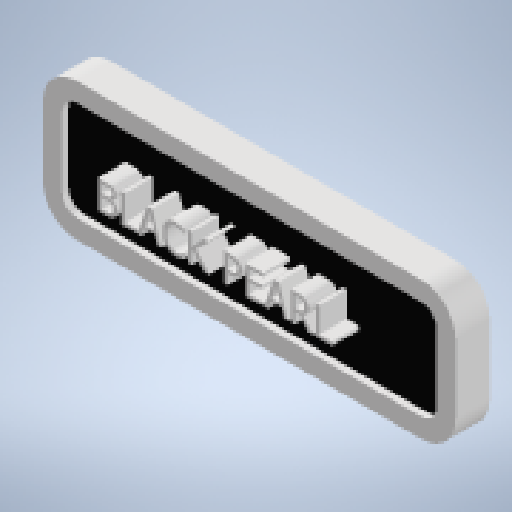
# Autodesk Inventor part: name of ship
Saved by Autodesk Inventor 2024.1 (Build 281209000, 209)
## iProperties
Created: 2023-10-19
Part Number: name of ship
Material: Generic
Document SubType Name: Modeling
Designer: Manaswi
Density: 1 g/cm^3
Appearance: Default
Author: Manaswi
Autodesk Inventor part; units mm, degrees
ref_plane "YZ Plane" through (0, 0, 0) normal (1, 0, 0) x (0, 1, 0)
ref_plane "XZ Plane" through (0, 0, 0) normal (0, 1, 0) x (-1, 0, 0)
ref_plane "XY Plane" through (0, 0, 0) normal (0, 0, 1) x (1, 0, 0)
sketch "Sketch1" plane through (0, 0, 0) normal (0, 0, 1) x (1, 0, 0)
  line L0 (0, 0) -> (6000, 0)
  line L1 (6000, 0) -> (6000, 2000)
  line L2 (6000, 2000) -> (0, 2000)
  line L3 (0, 2000) -> (0, 0)
  dimension "d0" = 2000
  dimension "d1" = 6000
  constraints: 8 end point, 3 perpendicular, 1 horizontal
  measures "d0" distance of L0.start L2.end
  measures "d1" distance of L2.end L1.end
extrude "Extrusion1" add sketch "Sketch1" along normal blind 500
fillet "Fillet1" radius 500 4 edges at (6000, 2000, 250) (6000, 0, 250) (0, 2000, 250) (0, 0, 250)
sketch "Sketch2" plane through (0, 0, 500) normal (0, 0, 1) x (1, 0, 0)
  arc A0 (0, 500) -> (500, 0) centre (500, 500) ccw projected
  line L0 (500, 0) -> (5500, 0) projected
  arc A1 (5500, 0) -> (6000, 500) centre (5500, 500) ccw projected
  line L1 (6000, 500) -> (6000, 1500) projected
  arc A2 (6000, 1500) -> (5500, 2000) centre (5500, 1500) ccw projected
  line L2 (5500, 2000) -> (500, 2000) projected
  arc A3 (500, 2000) -> (0, 1500) centre (500, 1500) ccw projected
  line L3 (0, 1500) -> (0, 500) projected
  line L4 (500, 1720.5162) -> (5500, 1720.5162)
  arc A4 (5720.5162, 1500) -> (5500, 1720.5162) centre (5500, 1500) ccw
  line L5 (5720.5162, 1500) -> (5720.5162, 500)
  arc A5 (5500, 279.4838) -> (5720.5162, 500) centre (5500, 500) ccw
  line L6 (5500, 279.4838) -> (500, 279.4838)
  arc A6 (279.4838, 500) -> (500, 279.4838) centre (500, 500) ccw
  line L7 (279.4838, 500) -> (279.4838, 1500)
  arc A7 (500, 1720.5162) -> (279.4838, 1500) centre (500, 1500) ccw
  point P0 (0, 0)
  constraints: 8 end point, 8 point on circle, 4 centre point, 7 other
extrude "Extrusion2" cut sketch "Sketch2" against normal blind 100 contours L4 A4 L5 A5 L6 A6 L7 A7
sketch "Sketch3" plane through (0, 0, 400) normal (0, 0, 1) x (1, 0, 0)
  line L0 (1060.4383, 1242.6804) -> (4504.2158, 1242.6804) construction
  line L1 (4504.2158, 1242.6804) -> (4504.2158, 811.7024) construction
  line L2 (4504.2158, 811.7024) -> (1060.4383, 811.7024) construction
  line L3 (1060.4383, 811.7024) -> (1060.4383, 1242.6804) construction
  spline S0 degree 2 poles (1384.8522, 946.931) (1384.8522, 915.906) (1361.2462, 868.3567) (1341.6869, 852.8442) knots 0 0 0 1 2 2 2
  spline S1 degree 2 poles (1341.6869, 852.8442) (1318.0809, 834.6339) (1264.4616, 819.1214) (1221.9708, 819.1214) knots 0 0 0 1 2 2 2
  line L4 (1221.9708, 819.1214) -> (1102.5919, 819.1214)
  line L5 (1102.5919, 819.1214) -> (1102.5919, 1235.2614)
  line L6 (1102.5919, 1235.2614) -> (1212.8656, 1235.2614)
  spline S2 degree 2 poles (1212.8656, 1235.2614) (1257.3798, 1235.2614) (1301.894, 1229.5285) (1322.1277, 1218.3999) knots 0 0 0 1 2 2 2
  spline S3 degree 2 poles (1322.1277, 1218.3999) (1344.722, 1206.5969) (1365.2929, 1167.8157) (1365.2929, 1141.5118) knots 0 0 0 1 2 2 2
  spline S4 degree 2 poles (1365.2929, 1141.5118) (1365.2929, 1112.173) (1334.2679, 1065.6354) (1306.9524, 1052.4835) knots 0 0 0 1 2 2 2
  line L7 (1306.9524, 1052.4835) -> (1306.9524, 1050.4601)
  spline S5 degree 2 poles (1306.9524, 1050.4601) (1344.0475, 1040.3433) (1384.8522, 986.7239) (1384.8522, 946.931) knots 0 0 0 1 2 2 2
  spline S6 degree 2 poles (1327.1861, 944.5704) (1327.1861, 968.1764) (1313.697, 998.5269) (1293.4633, 1009.3183) knots 0 0 0 1 2 2 2
  spline S7 degree 2 poles (1293.4633, 1009.3183) (1280.3113, 1016.0628) (1249.2863, 1020.1096) (1220.6219, 1020.1096) knots 0 0 0 1 2 2 2
  line L8 (1220.6219, 1020.1096) -> (1157.8974, 1020.1096)
  line L9 (1157.8974, 1020.1096) -> (1157.8974, 866.3334)
  line L10 (1157.8974, 866.3334) -> (1202.7488, 866.3334)
  spline S8 degree 2 poles (1202.7488, 866.3334) (1239.1695, 866.3334) (1280.9858, 873.0779) (1297.1728, 883.8693) knots 0 0 0 1 2 2 2
  spline S9 degree 2 poles (1297.1728, 883.8693) (1312.6853, 894.9978) (1327.1861, 922.6505) (1327.1861, 944.5704) knots 0 0 0 1 2 2 2
  spline S10 degree 2 poles (1307.6268, 1133.7556) (1307.6268, 1148.5936) (1297.51, 1170.8507) (1286.3815, 1177.2581) knots 0 0 0 1 2 2 2
  spline S11 degree 2 poles (1286.3815, 1177.2581) (1272.8923, 1184.6771) (1240.1811, 1188.0494) (1210.8423, 1188.0494) knots 0 0 0 1 2 2 2
  line L11 (1210.8423, 1188.0494) -> (1157.8974, 1188.0494)
  line L12 (1157.8974, 1188.0494) -> (1157.8974, 1066.3099)
  line L13 (1157.8974, 1066.3099) -> (1220.6219, 1066.3099)
  spline S12 degree 2 poles (1220.6219, 1066.3099) (1246.5885, 1066.3099) (1271.2062, 1071.7055) (1284.3581, 1080.1362) knots 0 0 0 1 2 2 2
  spline S13 degree 2 poles (1284.3581, 1080.1362) (1297.1728, 1088.2297) (1307.6268, 1114.1963) (1307.6268, 1133.7556) knots 0 0 0 1 2 2 2
  line L14 (1680.9388, 819.1214) -> (1439.8204, 819.1214)
  line L15 (1439.8204, 819.1214) -> (1439.8204, 1235.2614)
  line L16 (1439.8204, 1235.2614) -> (1495.1259, 1235.2614)
  line L17 (1495.1259, 1235.2614) -> (1495.1259, 868.3567)
  line L18 (1495.1259, 868.3567) -> (1680.9388, 868.3567)
  line L19 (1680.9388, 868.3567) -> (1680.9388, 819.1214)
  line L20 (1679.5899, 819.1214) -> (1819.877, 1235.2614)
  line L21 (1819.877, 1235.2614) -> (1887.9971, 1235.2614)
  line L22 (1887.9971, 1235.2614) -> (2028.2842, 819.1214)
  line L23 (2028.2842, 819.1214) -> (1969.9436, 819.1214)
  line L24 (1969.9436, 819.1214) -> (1932.1741, 935.4652)
  line L25 (1932.1741, 935.4652) -> (1773.3394, 935.4652)
  line L26 (1773.3394, 935.4652) -> (1735.5698, 819.1214)
  line L27 (1735.5698, 819.1214) -> (1679.5899, 819.1214)
  line L28 (1916.9988, 982.6772) -> (1852.5881, 1178.607)
  line L29 (1852.5881, 1178.607) -> (1788.5147, 982.6772)
  line L30 (1788.5147, 982.6772) -> (1916.9988, 982.6772)
  spline S14 degree 2 poles (2230.2841, 811.7024) (2189.8166, 811.7024) (2121.3592, 839.0179) (2096.4043, 866.3334) knots 0 0 0 1 2 2 2
  spline S15 degree 2 poles (2096.4043, 866.3334) (2071.4494, 893.3117) (2044.1339, 974.2465) (2044.1339, 1026.8541) knots 0 0 0 1 2 2 2
  spline S16 degree 2 poles (2044.1339, 1026.8541) (2044.1339, 1079.1246) (2070.775, 1156.6871) (2096.0671, 1185.3515) knots 0 0 0 1 2 2 2
  spline S17 degree 2 poles (2096.0671, 1185.3515) (2121.022, 1213.3415) (2189.1422, 1242.6804) (2231.2957, 1242.6804) knots 0 0 0 1 2 2 2
  spline S18 degree 2 poles (2231.2957, 1242.6804) (2252.2039, 1242.6804) (2288.9618, 1236.6103) (2304.4743, 1231.8891) knots 0 0 0 1 2 2 2
  spline S19 degree 2 poles (2304.4743, 1231.8891) (2317.9635, 1227.5051) (2345.9534, 1215.0277) (2359.7798, 1207.6086) knots 0 0 0 1 2 2 2
  line L31 (2359.7798, 1207.6086) -> (2359.7798, 1140.8374)
  line L32 (2359.7798, 1140.8374) -> (2355.3958, 1140.8374)
  spline S20 degree 2 poles (2355.3958, 1140.8374) (2347.9768, 1147.5819) (2325.0453, 1166.4667) (2308.5211, 1175.5719) knots 0 0 0 1 2 2 2
  spline S21 degree 2 poles (2308.5211, 1175.5719) (2292.6713, 1184.3399) (2255.239, 1195.4684) (2230.9585, 1195.4684) knots 0 0 0 1 2 2 2
  spline S22 degree 2 poles (2230.9585, 1195.4684) (2204.3175, 1195.4684) (2156.7682, 1173.5485) (2138.8951, 1152.6404) knots 0 0 0 1 2 2 2
  spline S23 degree 2 poles (2138.8951, 1152.6404) (2121.3592, 1131.395) (2101.8, 1066.9843) (2101.8, 1026.8541) knots 0 0 0 1 2 2 2
  spline S24 degree 2 poles (2101.8, 1026.8541) (2101.8, 984.0261) (2122.3709, 922.3133) (2140.244, 901.0679) knots 0 0 0 1 2 2 2
  spline S25 degree 2 poles (2140.244, 901.0679) (2157.7799, 880.497) (2204.6547, 859.5888) (2230.9585, 859.5888) knots 0 0 0 1 2 2 2
  spline S26 degree 2 poles (2230.9585, 859.5888) (2254.9017, 859.5888) (2295.7064, 871.3918) (2311.5561, 880.1597) knots 0 0 0 1 2 2 2
  spline S27 degree 2 poles (2311.5561, 880.1597) (2326.7314, 888.9277) (2349.3257, 907.138) (2355.7331, 913.5454) knots 0 0 0 1 2 2 2
  line L33 (2355.7331, 913.5454) -> (2359.7798, 913.5454)
  line L34 (2359.7798, 913.5454) -> (2359.7798, 847.4486)
  spline S28 degree 2 poles (2359.7798, 847.4486) (2345.9534, 841.0412) (2321.673, 829.2382) (2304.4743, 823.8426) knots 0 0 0 1 2 2 2
  spline S29 degree 2 poles (2304.4743, 823.8426) (2286.264, 817.7725) (2255.239, 811.7024) (2230.2841, 811.7024) knots 0 0 0 1 2 2 2
  line L35 (2714.8814, 819.1214) -> (2643.0518, 819.1214)
  line L36 (2643.0518, 819.1214) -> (2490.9617, 1012.6905)
  line L37 (2490.9617, 1012.6905) -> (2466.6812, 985.375)
  line L38 (2466.6812, 985.375) -> (2466.6812, 819.1214)
  line L39 (2466.6812, 819.1214) -> (2411.3758, 819.1214)
  line L40 (2411.3758, 819.1214) -> (2411.3758, 1235.2614)
  line L41 (2411.3758, 1235.2614) -> (2466.6812, 1235.2614)
  line L42 (2466.6812, 1235.2614) -> (2466.6812, 1044.0528)
  line L43 (2466.6812, 1044.0528) -> (2637.3189, 1235.2614)
  line L44 (2637.3189, 1235.2614) -> (2704.7646, 1235.2614)
  line L45 (2704.7646, 1235.2614) -> (2532.4408, 1049.4485)
  line L46 (2532.4408, 1049.4485) -> (2714.8814, 819.1214)
  spline S30 degree 2 poles (3189.6992, 1109.8124) (3189.6992, 1082.8341) (3170.4771, 1034.2732) (3153.2785, 1017.4117) knots 0 0 0 1 2 2 2
  spline S31 degree 2 poles (3153.2785, 1017.4117) (3131.6959, 996.1663) (3073.3553, 974.2465) (3028.8412, 974.2465) knots 0 0 0 1 2 2 2
  line L47 (3028.8412, 974.2465) -> (2981.9664, 974.2465)
  line L48 (2981.9664, 974.2465) -> (2981.9664, 819.1214)
  line L49 (2981.9664, 819.1214) -> (2926.6609, 819.1214)
  line L50 (2926.6609, 819.1214) -> (2926.6609, 1235.2614)
  line L51 (2926.6609, 1235.2614) -> (3031.2018, 1235.2614)
  spline S32 degree 2 poles (3031.2018, 1235.2614) (3068.2969, 1235.2614) (3120.2301, 1223.1211) (3140.1266, 1209.2948) knots 0 0 0 1 2 2 2
  spline S33 degree 2 poles (3140.1266, 1209.2948) (3163.3954, 1193.445) (3189.6992, 1144.5469) (3189.6992, 1109.8124) knots 0 0 0 1 2 2 2
  spline S34 degree 2 poles (3132.0331, 1108.1262) (3132.0331, 1129.7088) (3117.195, 1161.4083) (3102.0198, 1171.5252) knots 0 0 0 1 2 2 2
  spline S35 degree 2 poles (3102.0198, 1171.5252) (3088.8678, 1180.2931) (3053.7961, 1187.3749) (3027.8295, 1187.3749) knots 0 0 0 1 2 2 2
  line L52 (3027.8295, 1187.3749) -> (2981.9664, 1187.3749)
  line L53 (2981.9664, 1187.3749) -> (2981.9664, 1021.4585)
  line L54 (2981.9664, 1021.4585) -> (3019.736, 1021.4585)
  spline S36 degree 2 poles (3019.736, 1021.4585) (3053.4589, 1021.4585) (3094.938, 1032.2498) (3108.4271, 1046.4134) knots 0 0 0 1 2 2 2
  spline S37 degree 2 poles (3108.4271, 1046.4134) (3120.9046, 1058.8909) (3132.0331, 1088.2297) (3132.0331, 1108.1262) knots 0 0 0 1 2 2 2
  line L55 (3242.3068, 819.1214) -> (3242.3068, 1235.2614)
  line L56 (3242.3068, 1235.2614) -> (3502.6472, 1235.2614)
  line L57 (3502.6472, 1235.2614) -> (3502.6472, 1186.026)
  line L58 (3502.6472, 1186.026) -> (3297.6123, 1186.026)
  line L59 (3297.6123, 1186.026) -> (3297.6123, 1072.0428)
  line L60 (3297.6123, 1072.0428) -> (3488.8209, 1072.0428)
  line L61 (3488.8209, 1072.0428) -> (3488.8209, 1022.8074)
  line L62 (3488.8209, 1022.8074) -> (3297.6123, 1022.8074)
  line L63 (3297.6123, 1022.8074) -> (3297.6123, 868.3567)
  line L64 (3297.6123, 868.3567) -> (3502.6472, 868.3567)
  line L65 (3502.6472, 868.3567) -> (3502.6472, 819.1214)
  line L66 (3502.6472, 819.1214) -> (3242.3068, 819.1214)
  line L67 (3518.497, 819.1214) -> (3658.784, 1235.2614)
  line L68 (3658.784, 1235.2614) -> (3726.9042, 1235.2614)
  line L69 (3726.9042, 1235.2614) -> (3867.1913, 819.1214)
  line L70 (3867.1913, 819.1214) -> (3808.8507, 819.1214)
  line L71 (3808.8507, 819.1214) -> (3771.0811, 935.4652)
  line L72 (3771.0811, 935.4652) -> (3612.2465, 935.4652)
  line L73 (3612.2465, 935.4652) -> (3574.4769, 819.1214)
  line L74 (3574.4769, 819.1214) -> (3518.497, 819.1214)
  line L75 (3755.9058, 982.6772) -> (3691.4952, 1178.607)
  line L76 (3691.4952, 1178.607) -> (3627.4218, 982.6772)
  line L77 (3627.4218, 982.6772) -> (3755.9058, 982.6772)
  line L78 (4228.7002, 819.1214) -> (4156.8705, 819.1214)
  line L79 (4156.8705, 819.1214) -> (4025.3514, 984.7006)
  line L80 (4025.3514, 984.7006) -> (3961.9525, 984.7006)
  line L81 (3961.9525, 984.7006) -> (3961.9525, 819.1214)
  line L82 (3961.9525, 819.1214) -> (3906.647, 819.1214)
  line L83 (3906.647, 819.1214) -> (3906.647, 1235.2614)
  line L84 (3906.647, 1235.2614) -> (4013.8857, 1235.2614)
  spline S38 degree 2 poles (4013.8857, 1235.2614) (4049.6319, 1235.2614) (4097.8556, 1227.5051) (4119.7754, 1213.3415) knots 0 0 0 1 2 2 2
  spline S39 degree 2 poles (4119.7754, 1213.3415) (4141.6953, 1199.1779) (4166.9874, 1155.001) (4166.9874, 1122.2898) knots 0 0 0 1 2 2 2
  spline S40 degree 2 poles (4166.9874, 1122.2898) (4166.9874, 1076.764) (4120.4499, 1015.0511) (4080.6569, 1000.2131) knots 0 0 0 1 2 2 2
  line L85 (4080.6569, 1000.2131) -> (4228.7002, 819.1214)
  spline S41 degree 2 poles (4109.3213, 1117.9058) (4109.3213, 1136.1162) (4096.5066, 1164.1061) (4083.0175, 1173.2113) knots 0 0 0 1 2 2 2
  spline S42 degree 2 poles (4083.0175, 1173.2113) (4071.2145, 1180.9676) (4039.8523, 1187.3749) (4016.9207, 1187.3749) knots 0 0 0 1 2 2 2
  line L86 (4016.9207, 1187.3749) -> (3961.9525, 1187.3749)
  line L87 (3961.9525, 1187.3749) -> (3961.9525, 1030.9009)
  line L88 (3961.9525, 1030.9009) -> (4010.5134, 1030.9009)
  spline S43 degree 2 poles (4010.5134, 1030.9009) (4034.4566, 1030.9009) (4072.5634, 1039.3316) (4085.7153, 1052.4835) knots 0 0 0 1 2 2 2
  spline S44 degree 2 poles (4085.7153, 1052.4835) (4097.8556, 1063.9493) (4109.3213, 1096.3232) (4109.3213, 1117.9058) knots 0 0 0 1 2 2 2
  line L89 (4502.867, 819.1214) -> (4261.7486, 819.1214)
  line L90 (4261.7486, 819.1214) -> (4261.7486, 1235.2614)
  line L91 (4261.7486, 1235.2614) -> (4317.0541, 1235.2614)
  line L92 (4317.0541, 1235.2614) -> (4317.0541, 868.3567)
  line L93 (4317.0541, 868.3567) -> (4502.867, 868.3567)
  line L94 (4502.867, 868.3567) -> (4502.867, 819.1214)
  point P0 (0, 0)
  constraints: 2 other
extrude "Extrusion3" add sketch "Sketch3" along normal blind 400
body "Solid1"
